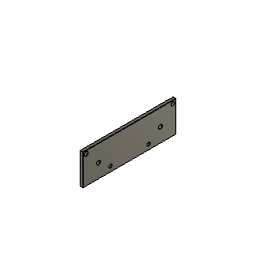
Plate2 (Autodesk Fusion 360 design; units mm, degrees)
Autodesk Fusion 360 part; units mm, degrees
sketch "Sketch1" plane through (13.4, 0, 0) normal (1, 0, 0) x (0, 1, 0)
  circle A0 centre (3, 27) radius 1.75
  line L0 (0, 0) -> (90, 0)
  line L1 (90, 0) -> (90, 30)
  line L2 (90, 30) -> (0, 30)
  line L3 (0, 30) -> (0, 0)
  circle A1 centre (3, 27) radius 1.75
  circle A2 centre (87, 27) radius 1.75
  line L4 (0, 13.75) -> (90, 13.75) construction
  circle A3 centre (15, 13.75) radius 1.75
  circle A4 centre (75, 13.75) radius 1.75
  line L5 (0, 5) -> (90, 5) construction
  circle A5 centre (26.5, 5) radius 1.4
  circle A6 centre (63.5, 5) radius 1.4
  circle A7 centre (3, 27) radius 2.9
  dimension "d24" = 3.5
  dimension "d25" = 3
  dimension "d26" = 3
  dimension "d27" = 3.5
  dimension "d28" = 3.5
  dimension "d29" = 16.25
  dimension "d30" = 30
  dimension "d31" = 15
  dimension "d32" = 60
  dimension "d33" = 2.8
  dimension "d34" = 2.8
  dimension "d35" = 25
  dimension "d36" = 26.5
  dimension "d37" = 37
  constraint horizontal L0
  constraint vertical L1
  constraint horizontal L2
  constraint vertical L3
  constraint coincident L0.start L3.end
  constraint coincident L3 L4.start
  constraint coincident L1 L4.end
  constraint perpendicular L1 L4
  constraint coincident L4 A3.centre
  constraint coincident L4 A4.centre
  constraint coincident L3 L5.start
  constraint coincident L1 L5.end
  constraint perpendicular L1 L5
  constraint coincident L5 A5.centre
  constraint coincident L5 A6.centre
  measures "d24" diameter of A2
  measures "d25" distance of L2 A2.centre
  measures "d26" distance of L1 A2.centre
  measures "d27" diameter of A3
  measures "d28" diameter of A4
  measures "d29" distance of L2 L4
  measures "d30" distance of L0 L2
  measures "d31" distance of L3 A3.centre
  measures "d32" distance of A3.centre A4.centre
  measures "d33" diameter of A5
  measures "d34" diameter of A6
  measures "d35" distance of L2 L5
  measures "d36" distance of L3 A5.centre
  measures "d37" distance of A5.centre A6.centre
extrude "Extrude1" add sketch "Sketch1" along normal blind 3 contours L0 L1 L2 L3 | A7
chamfer "Chamfer1" distance 0.2 angle 45 8 edges at (13.4, 45, 30) (16.4, 45, 30) (16.4, 0, 15) (13.4, 0, 15) (16.4, 45, 0) (13.4, 45, 0) (13.4, 90, 15) (16.4, 90, 15)
chamfer "Chamfer1" distance 0.2 angle 45 4 edges at (16.4, 73.3684, 14.3828) (16.4, 13.3684, 14.3828) (16.4, 25.1947, 5.5063) (16.4, 62.1947, 5.5063)
chamfer "Chamfer1" distance 0.2 angle 45 4 edges at (13.4, 13.3684, 14.3828) (13.4, 25.1947, 5.5063) (13.4, 62.1947, 5.5063) (13.4, 73.3684, 14.3828)
chamfer "Chamfer1" distance 0.2 angle 45 1 edges at (16.4, 1.3684, 27.6328)
